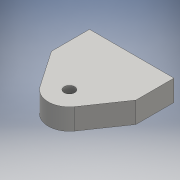
# Autodesk Inventor part: chuck support
Saved by Autodesk Inventor 2016 SP1 (Build 200210100, 210)
## iProperties
Created: 2016-05-26
Part Number: chuck support
Material: Generic
Document SubType Name: Modeling
Designer: ubik
Density: 1 g/cm^3
Appearance: Default
Author: ubik
Autodesk Inventor part; units mm, degrees
ref_plane "YZ Plane" through (0, 0, 0) normal (1, 0, 0) x (0, 1, 0)
ref_plane "XZ Plane" through (0, 0, 0) normal (0, 1, 0) x (-1, 0, 0)
ref_plane "XY Plane" through (0, 0, 0) normal (0, 0, 1) x (1, 0, 0)
sketch "Sketch1" plane through (0, 0, 0) normal (0, 0, 1) x (1, 0, 0)
  circle A0 centre (0, 0) radius 2.5
  line L0 (-20, 29.5) -> (20, 29.5)
  circle A1 centre (0, 0) radius 10
  line L1 (20, 29.5) -> (20, 11.5)
  line L2 (20, 11.5) -> (8.2497, -5.6517)
  line L3 (-20, 29.5) -> (-20, 11.5)
  line L4 (-20, 11.5) -> (-8.2497, -5.6517)
  dimension "d0" = 5
  dimension "d1" = 29.5
  dimension "d2" = 40
  dimension "d3" = 20
  dimension "d4" = 18
  dimension "d5" = 20
  constraints: 10 end point, 2 centre point, 2 coincident, 2 point on circle, 2 tangent, 2 vertical, 1 horizontal
  measures "d0" diameter of A0
  measures "d1" distance from line of point (0, 0) L0
  measures "d2" distance of L0.start L0.end
  measures "d3" diameter of A1
  measures "d4" distance of L0.end L1.end
  measures "d5" distance from line of point (0, 0) L3
extrude "Extrusion1" add sketch "Sketch1" along normal blind 10
equation "\"d5\" = 0.5 * d2"
body "Solid1"
